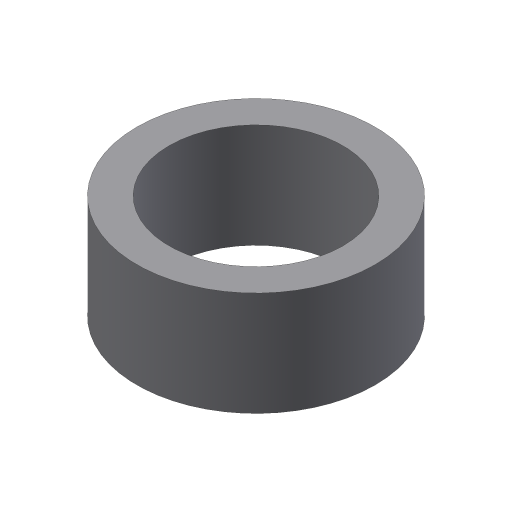
# Autodesk Inventor part: Federteller
Saved by Autodesk Inventor 2023 (Build 270158000, 158)
## iProperties
Created: 2025-01-21
Part Number: Federteller
Material: Generisch
Document SubType Name: Modeling
Designer: abdel
Density: 1 g/cm^3
Appearance: Vorgabe
Author: abdel
Autodesk Inventor part; units mm, degrees
ref_plane "YZ Plane" through (0, 0, 0) normal (1, 0, 0) x (0, 1, 0)
ref_plane "XZ Plane" through (0, 0, 0) normal (0, 1, 0) x (-1, 0, 0)
ref_plane "XY Plane" through (0, 0, 0) normal (0, 0, 1) x (1, 0, 0)
sketch "Skizze1" plane through (0, 0, 0) normal (0, 0, 1) x (1, 0, 0)
  circle A0 centre (0, 0) radius 6
  circle A1 centre (0, 0) radius 4.375
  dimension "d0" = 12
  dimension "d6" = 8.75
  constraints: 2 centre point, 2 coincident
  measures "d0" diameter of A0
  measures "d6" diameter of A1
extrude "Extrusion3" add sketch "Skizze1" along normal blind 5.25
